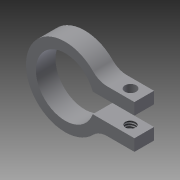
# Autodesk Inventor part: bearing_blcok
Saved by Autodesk Inventor 2013 (Build 170138000, 138)
## iProperties
Created: 2013-09-17
Part Number: bearing_blcok
Material: Generic
Document SubType Name: Modeling
Designer: Ian
Density: 1 g/cm^3
Mass: 1.75864 g
Surface Area: 17.3763 cm^2
Volume: 1.75864 cm^3
Author: Ian
Autodesk Inventor part; units mm, degrees
note: some values were not read from the file. Chosen so that the rebuilt part matches the saved one: direction of "Hole1"; direction of "Hole2".
ref_plane "YZ Plane" through (0, 0, 0) normal (1, 0, 0) x (0, 1, 0)
ref_plane "XZ Plane" through (0, 0, 0) normal (0, 1, 0) x (-1, 0, 0)
ref_plane "XY Plane" through (0, 0, 0) normal (0, 0, 1) x (1, 0, 0)
sketch "Sketch1" plane through (0, 0, 0) normal (0, 0, 1) x (1, 0, 0)
  arc A0 (8.9398, 3.175) -> (8.9398, -3.175) centre (0, 0) ccw
  arc A1 (9.0696, 8.89) -> (9.0696, -8.89) centre (0, 0) ccw
  line L0 (8.9398, 3.175) -> (12.2967, 3.175)
  line L1 (8.9398, -3.175) -> (12.2967, -3.175)
  line L2 (12.2967, 3.175) -> (22.4567, 3.175)
  line L3 (12.2967, -3.175) -> (22.4567, -3.175)
  line L4 (22.4567, 3.175) -> (22.4567, 6.985)
  line L5 (22.4567, 6.985) -> (13.6044, 6.985)
  line L6 (22.4567, -3.175) -> (22.4567, -6.985)
  line L7 (22.4567, -6.985) -> (13.6044, -6.985)
  line L8 (-18.034, 0) -> (28.275, 0) construction
  arc A2 (9.0696, 8.89) -> (13.6044, 6.985) centre (13.6044, 13.335) ccw
  arc A3 (13.6044, -6.985) -> (9.0696, -8.89) centre (13.6044, -13.335) ccw
  point P0 (10.6066, 6.985)
  point P1 (10.6066, -6.985)
  dimension "d0" = 18.9738
  dimension "d1" = 25.4
  dimension "d8" = 3.81
  dimension "d18" = 3.175
  dimension "d19" = 6.35
  dimension "d20" = 13.5169
  dimension "d21" = 8.8523
  constraints: 18 end point, 12 point on circle, 4 centre point, 4 perpendicular, 4 tangent, 3 parallel, 2 coincident, 2 horizontal, 2 point on line, 1 equal radius, 1 symmetric about line, 3 other
  measures "d0" diameter of A0
  measures "d1" diameter of A1
  measures "d8" distance of L2.end L4.end
  measures "d18" distance from line of L0 point (0, 0)
  measures "d19" radius of A2
  measures "d20" distance of L2.end L0.start
  measures "d21" distance of L4.end L5.end
extrude "Extrusion1" add sketch "Sketch1" along normal blind 6.35
sketch "Sketch2" plane through (13.6044, 6.985, 0) normal (0, 1, 0) x (1, 0, 0)
  line L0 (0, 0) -> (8.8523, 0) projected
  line L1 (8.8523, -6.35) -> (0, -6.35) projected
  line L2 (4.4262, -6.35) -> (4.4262, 0) construction
  point P0 (-13.6044, 0)
  point P1 (4.4262, -3.175)
  constraints: 3 midpoint, 2 end point
hole "Hole1" at (18.0306, 6.985, 3.175) direction (0, -1, 0) diameter 3.6576 end up to surface clearance for "Flat Head Machine Screw (82)" size "#6" standard "Ansi Unified Screw Threads"
sketch "Sketch3" plane through (13.6044, -6.985, 0) normal (0, -1, 0) x (1, 0, 0)
  circle A0 centre (4.4262, 3.175) radius 1.8288 projected
  point P0 (-13.6044, 0)
hole "Hole2" at (18.0306, -6.985, 3.175) direction (0, 1, 0) diameter 3.302 end up to surface thread size "8-32 UNC" class "2B" standard "ANSI Unified Screw Threads"
body "Solid1"
